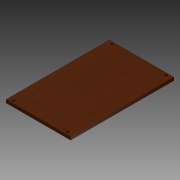
# Autodesk Inventor part: two_part_wastebaord
Saved by Autodesk Inventor 2014 (Build 180170000, 170)
## iProperties
Created: 2013-07-16
Part Number: two_part_wastebaord
Material: Wood (Walnut)
Document SubType Name: Modeling
Designer: Edward
Density: 0.55 g/cm^3
Appearance: Walnut - Natural Polished
Author: Edward
Autodesk Inventor part; units mm, degrees
ref_plane "YZ Plane" through (0, 0, 0) normal (1, 0, 0) x (0, 1, 0)
ref_plane "XZ Plane" through (0, 0, 0) normal (0, 1, 0) x (-1, 0, 0)
ref_plane "XY Plane" through (0, 0, 0) normal (0, 0, 1) x (1, 0, 0)
sketch "Sketch1" plane through (0, 0, 0) normal (0, 0, 1) x (1, 0, 0)
  line L0 (-125, 200) -> (125, 200)
  line L1 (125, 200) -> (125, -200)
  line L2 (125, -200) -> (-125, -200)
  line L3 (-125, -200) -> (-125, 200)
  point P0 (0, 0)
  dimension "d0" = 250
  dimension "d1" = 400
  dimension "d2" = 125
  dimension "d3" = 200
  constraints: 8 end point, 2 parallel, 1 horizontal, 1 perpendicular
  measures "d0" distance of L1.end L2.end
  measures "d1" distance of L0.end L1.end
  measures "d2" distance from line of point (0, 0) L3
  measures "d3" distance from line of L0 point (0, 0)
extrude "Extrusion1" add sketch "Sketch1" along normal blind 12.7
sketch "Sketch2" plane through (0, 0, 12.7) normal (0, 0, 1) x (1, 0, 0)
  line L0 (-125, -200) -> (125, -200) projected
  line L1 (125, -200) -> (125, 200) projected
  circle A0 centre (105, -190) radius 2.75
  point P0 (0, 0)
  dimension "d6" = 5.5
  dimension "d7" = 10
  dimension "d8" = 20
  constraints: 1 centre point
  measures "d6" diameter of A0
  measures "d7" distance from line of L0 A0.centre
  measures "d8" distance from line of L1 A0.centre
hole "Hole1" at (105, -190, 12.7) direction (0, 0, -1) diameter 5 end through all counterbore diameter 11 counterbore depth 6
pattern_linear "Rectangular Pattern1" count 2 spacing 210 along (-1, 0, 0) count 2 spacing 380 along (0, 1, 0) of "Hole1"
equation "\"d2\" = 0.5 * d0"
equation "\"d3\" = 0.5 * d1"
body "Solid1"
